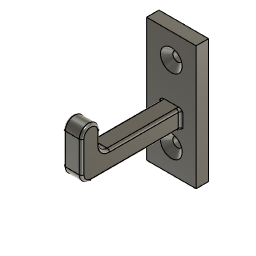
exampleHook v1 (Autodesk Fusion 360 design; units mm, degrees)
Autodesk Fusion 360 part; units mm, degrees
sketch "Sketch1" plane through (0, 0, 0) normal (0, 1, 0) x (1, 0, 0) in component "Component"
  line L0 (12.7, 31.75) -> (-12.7, 31.75)
  line L1 (-12.7, 31.75) -> (-12.7, -31.75)
  line L2 (-12.7, -31.75) -> (12.7, -31.75)
  line L3 (12.7, -31.75) -> (12.7, 31.75)
  line L4 (12.7, 31.75) -> (-12.7, -31.75) construction
  line L5 (-12.7, 31.75) -> (12.7, -31.75) construction
  dimension "d1" = 63.5
  dimension "d2" = 25.4
  constraint perpendicular L0 L1
  constraint parallel L0 L2
  constraint parallel L1 L3
  constraint horizontal L0
  constraint coincident L4 origin
  constraint coincident L5 origin
  measures "d1" distance of L0.start L2.end
  measures "d2" distance of L1.end L2.end
extrude "Extrude1" add sketch "Sketch1" along normal blind 6.35 in component "Component"
hole "Hole1" at (0, 0, 19.05) direction (0, 1, 0) diameter 4.826 end through all in component "Component"
mirror "Mirror1" about plane through (0, 0, 0) normal (0, 0, 1) of "Hole1" in component "Component"
sketch "Sketch2" plane through (0, 0, 0) normal (1, 0, 0) x (0, 1, 0) in component "Component"
  line L0 (0, -9.525) -> (-50.8, -9.525)
  line L1 (-50.8, -9.525) -> (-50.8, 15.875)
  line L2 (-50.8, 15.875) -> (-41.275, 15.875)
  line L3 (-41.275, 15.875) -> (-41.275, 0)
  line L4 (-41.275, 0) -> (0, 0)
  line L5 (0, 0) -> (0, -9.525)
  line L6 (0, 0) -> (-81.1043, 0) construction
  dimension "d11" = 9.525
  dimension "d12" = 9.525
  dimension "d13" = 50.8
  dimension "d14" = 25.4
  constraint horizontal L0
  constraint perpendicular L0 L1
  constraint perpendicular L1 L2
  constraint perpendicular L2 L3
  constraint perpendicular L3 L4
  constraint perpendicular L0 L5
  constraint coincident L4.end L5.start
  constraint parallel L0 L6
  measures "d11" distance of L1.end L2.end
  measures "d12" distance of L0.start L4.end
  measures "d13" distance of L0.start L0.end
  measures "d14" distance of L0.end L1.end
extrude "Extrude2" add sketch "Sketch2" along normal mid plane 9.525 in component "Component"
fillet "Fillet1" radius 4.7625 4 edges at (0, -50.8, -9.525) (0, -41.275, 0) (0, -50.8, 15.875) (0, -41.275, 15.875) in component "Component"
fillet "Fillet2" radius 1.1906 14 edges at (4.7625, -18.2563, 0) (4.7625, -39.8801, 1.3949) (4.7625, -41.275, 7.9375) (4.7625, -46.0375, 15.875) (4.7625, -50.8, 3.175) (4.7625, -49.4051, -8.1301) (4.7625, -23.0187, -9.525) (-4.7625, -23.0187, -9.525) (-4.7625, -49.4051, -8.1301) (-4.7625, -50.8, 3.175) (-4.7625, -46.0375, 15.875) (-4.7625, -41.275, 7.9375) (-4.7625, -39.8801, 1.3949) (-4.7625, -18.2563, 0) in component "Component"
fillet "Fillet2" radius 1.1906 2 edges at (-4.7625, 0, -4.7625) (4.7625, 0, -4.7625) in component "Component"
chamfer "Chamfer1" distance 3.175 angle 45 2 edges at (0.8726, 0, 21.2997) (-0.8726, 0, -21.2997) in component "Component"
component "Component" placed x (1, 0, 0) y (0, 1, 0) z (0, 0, 1) at (0, 0, 0)
equation "d11 = ( 3 / 8 ) * 1 in"
equation "d15 = ( 3 / 8 ) * 1 in"
equation "d17 = ( 3 / 16 ) * 1 in"
equation "d18 = ( 3 / 64 ) * 1 in"
equation "d19 = ( 3 / 64 ) * 1 in"
